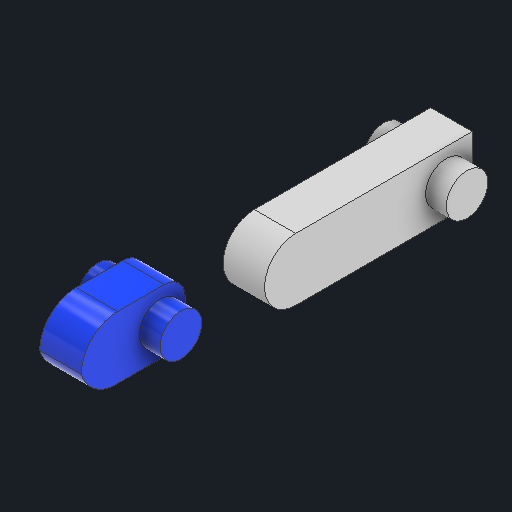
# Autodesk Inventor part: Part4final
Saved by Autodesk Inventor 2026 (Build 300175050, 175E)
## iProperties
Created: 2026-05-04
Part Number: Part4final
Material: Generic
Document SubType Name: Modeling
Designer: ptp527
Density: 1 g/cm^3
Appearance: Default
Author: ptp527
Autodesk Inventor part; units mm, degrees
ref_plane "YZ Plane" through (0, 0, 0) normal (1, 0, 0) x (0, 1, 0)
ref_plane "XZ Plane" through (0, 0, 0) normal (0, 1, 0) x (-1, 0, 0)
ref_plane "XY Plane" through (0, 0, 0) normal (0, 0, 1) x (1, 0, 0)
sketch "Sketch1" plane through (0, 0, 0) normal (0, 0, 1) x (1, 0, 0)
  line L0 (-20, -30) -> (20, -30)
  line L1 (20, -30) -> (20, 30)
  line L2 (20, 30) -> (-20, 30)
  line L3 (-20, 30) -> (-20, -30)
  line L4 (-20, -30) -> (20, 30) construction
  line L5 (20, -30) -> (-20, 30) construction
  point P0 (0, 0)
  dimension "d0" = 40
  dimension "d1" = 20
  dimension "d2" = 30
  constraints: 12 end point, 2 midpoint, 2 parallel, 1 horizontal, 1 perpendicular
  measures "d0" distance of L1.end L2.end
  measures "d1" distance from line of point (0, 0) L3
  measures "d2" distance from line of L2 point (0, 0)
extrude "Extrusion1" add sketch "Sketch1" along normal blind 100
sketch "Sketch2" plane through (20, -30, 0) normal (1, 0, 0) x (0, 0, -1)
  circle A0 centre (-24, 30) radius 20
  line L0 (0, 0) -> (0, 60) projected
  line L1 (0, 60) -> (-100, 60) projected
  point P0 (0, 30)
  point P1 (0, 30)
  dimension "d5" = 40
  dimension "d6" = 24
  dimension "d7" = 30
  constraints: 1 centre point, 1 midpoint
  measures "d5" diameter of A0
  measures "d6" distance of point (0, 30) A0.centre
  measures "d7" distance from line of L1 A0.centre
extrude "Extrusion2" add sketch "Sketch2" along normal blind 20 and the other way blind 20
sketch "Sketch3" plane through (-20, -30, 0) normal (-1, 0, 0) x (0, 0, 1)
  point P0 (0, 30)
sketch "Sketch4" plane through (-20, -30, 0) normal (-1, 0, 0) x (0, 0, 1)
  circle A0 centre (24, 30) radius 20 projected
  circle A1 centre (24, 30) radius 20
  line L0 (0, 60) -> (0, 0) projected
  point P0 (0, 30)
  point P1 (0, 30)
  dimension "d12" = 24
  constraints: 1 centre point, 1 coincident, 1 midpoint
  measures "d12" distance of point (0, 30) A1.centre
extrude "Extrusion3" add sketch "Sketch4" along normal blind 20 and the other way blind 20
fillet "Fillet1" radius 20 2 edges at (0, 30, 0) (0, -30, 0)
fillet "Fillet2" radius 35 2 edges at (0, 30, 100) (0, -30, 100)
sketch "Sketch5" plane through (20, -10, 0) normal (1, 0, 0) x (0, 0, -1)
  line L0 (236.5775, -0.6232) -> (36.5775, -0.6232)
  line L1 (36.5775, -0.6232) -> (36.5775, 59.3768)
  line L2 (36.5775, 59.3768) -> (236.5775, 59.3768)
  line L3 (236.5775, 59.3768) -> (236.5775, -0.6232)
  point P0 (0, 10)
  dimension "d19" = 60
  dimension "d20" = 200
  constraints: 8 end point, 2 parallel, 1 horizontal, 1 perpendicular
  measures "d19" distance of L0.end L1.end
  measures "d20" distance of L1.end L2.end
extrude "Extrusion4" add sketch "Sketch5" along normal blind 40
sketch "Sketch6" plane through (60, -10, 0) normal (1, 0, 0) x (0, 0, -1)
  circle A0 centre (211.5775, 29.3768) radius 20
  line L0 (236.5775, -0.6232) -> (236.5775, 59.3768) projected
  line L1 (236.5775, 59.3768) -> (36.5775, 59.3768) projected
  point P0 (0, 10)
  dimension "d23" = 40
  dimension "d24" = 25
  dimension "d25" = 30
  constraints: 1 centre point
  measures "d23" diameter of A0
  measures "d24" distance from line of L0 A0.centre
  measures "d25" distance from line of L1 A0.centre
extrude "Extrusion5" add sketch "Sketch6" along normal mid plane 40
sketch "Sketch7" plane through (20, -10, 0) normal (-1, 0, 0) x (0, 0, 1)
  circle A0 centre (-211.5775, 29.3768) radius 20 projected
  circle A1 centre (-211.5775, 29.3768) radius 20
  line L0 (-236.5775, -0.6232) -> (-236.5775, 59.3768) projected
  line L1 (-36.5775, -0.6232) -> (-236.5775, -0.6232) projected
  point P0 (0, 10)
  dimension "d28" = 40
  dimension "d29" = 25
  dimension "d30" = 30
  constraints: 1 centre point, 1 coincident
  measures "d28" diameter of A0
  measures "d29" distance from line of L0 A1.centre
  measures "d30" distance from line of L1 A1.centre
extrude "Extrusion6" add sketch "Sketch7" along normal mid plane 40
fillet "Fillet3" radius 30 2 edges at (40, 49.3768, -36.5775) (40, -10.6232, -36.5775)
body "Solid1"
